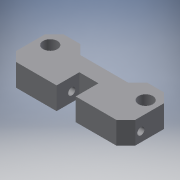
# Autodesk Inventor part: sensor bracket
Saved by Autodesk Inventor 2016 (Build 200138000, 138)
## iProperties
Created: 2016-01-06
Part Number: sensor bracket
Material: Generic
Document SubType Name: Modeling
Designer: RMcComber
Density: 1 g/cm^3
Appearance: Default
Author: RMcComber
Autodesk Inventor part; units mm, degrees
ref_plane "YZ Plane" through (0, 0, 0) normal (1, 0, 0) x (0, 1, 0)
ref_plane "XZ Plane" through (0, 0, 0) normal (0, 1, 0) x (-1, 0, 0)
ref_plane "XY Plane" through (0, 0, 0) normal (0, 0, 1) x (1, 0, 0)
sketch "Sketch1" plane through (0, 0, 0) normal (0, 0, 1) x (1, 0, 0)
  line L0 (0, 0) -> (60, 0) construction
  circle A0 centre (0, 0) radius 4.5
  circle A1 centre (60, 0) radius 4.5
  line L1 (67.5, -20) -> (-7.5, -20)
  line L2 (-7.5, -20) -> (-7.5, 20)
  line L3 (-7.5, 20) -> (67.5, 20)
  line L4 (67.5, 20) -> (67.5, -20)
  line L5 (67.5, -20) -> (-7.5, 20) construction
  line L6 (-7.5, -20) -> (67.5, 20) construction
  point P0 (30, 0)
  dimension "d0" = 9
  dimension "d1" = 60
  dimension "d2" = 40
  dimension "d3" = 75
  constraints: 14 end point, 3 midpoint, 2 centre point, 2 coincident, 2 horizontal, 2 parallel, 1 equal radius, 1 perpendicular
  measures "d0" diameter of A0
  measures "d1" distance of L0.start L0.end
  measures "d2" distance of L1.end L2.end
  measures "d3" distance of L2.end L3.end
extrude "Extrusion1" add sketch "Sketch1" along normal blind 14
sketch "Sketch2" plane through (0, 0, 14) normal (0, 0, 1) x (1, 0, 0)
  line L0 (-7.5, -20) -> (67.5, -20) projected
  line L1 (24, -20) -> (36, -20)
  line L2 (36, -20) -> (36, -5.7)
  line L3 (36, -5.7) -> (24, -5.7)
  line L4 (24, -5.7) -> (24, -20)
  point P0 (30, -20)
  dimension "d6" = 12
  dimension "d7" = 14.3
  constraints: 8 end point, 2 midpoint, 2 parallel, 1 horizontal, 1 perpendicular
  measures "d6" distance of L2.end L3.end
  measures "d7" distance of L3.end L1.start
extrude "Extrusion2" cut sketch "Sketch2" against normal through all
sketch "Sketch3" plane through (24, -20, 14) normal (1, 0, 0) x (0, 0, -1)
  line L0 (0, 0) -> (8, 0) construction
  line L1 (8, 0) -> (8, 9.5) construction
  line L2 (8, 9.5) -> (0, 9.5) construction
  line L3 (0, 9.5) -> (0, 0) construction
  circle A0 centre (8, 9.5) radius 2.25
  point P0 (14, 20)
  dimension "d10" = 8
  dimension "d11" = 9.5
  dimension "d12" = 4.5
  constraints: 8 end point, 2 parallel, 1 centre point, 1 coincident, 1 horizontal, 1 perpendicular
  measures "d10" distance of L1.end L2.end
  measures "d11" distance of L0.end L1.end
  measures "d12" diameter of A0
extrude "Extrusion3" cut sketch "Sketch3" along normal through all both and the other way through all
sketch "Sketch4" plane through (0, 0, 14) normal (0, 0, 1) x (1, 0, 0)
  line L0 (67.5, -20) -> (67.5, 20) projected
  circle A0 centre (0, 0) radius 4.5 projected
  line L1 (-7.5, 20) -> (67.5, 20)
  line L2 (67.5, 20) -> (67.5, 10)
  line L3 (67.5, 10) -> (-7.5, 10)
  line L4 (-7.5, 10) -> (-7.5, 20)
  dimension "d15" = 10
  constraints: 8 end point, 2 parallel, 1 horizontal, 1 perpendicular, 1 point on line
  measures "d15" distance from line of A0.centre L3
extrude "Extrusion4" cut sketch "Sketch4" against normal through all contours L3 L4 L1 L0
sketch "Sketch5" plane through (0, 0, 0) normal (0, 0, -1) x (-1, 0, 0)
  line L0 (7.5, 10) -> (-67.5, 10) projected
  line L1 (-45, 10) -> (-15, 10)
  line L2 (-15, 10) -> (-15, 4)
  line L3 (-15, 4) -> (-45, 4)
  line L4 (-45, 4) -> (-45, 10)
  point P0 (-30, 10)
  dimension "d18" = 30
  dimension "d19" = 6
  constraints: 8 end point, 2 midpoint, 2 parallel, 1 horizontal, 1 perpendicular
  measures "d18" distance of L2.end L3.end
  measures "d19" distance of L3.end L1.start
extrude "Extrusion5" cut sketch "Sketch5" against normal through all
chamfer "Chamfer1" distance 6 angle 45 2 edges at (45, 10, 7) (15, 10, 7)
chamfer "Chamfer2" distance 6 angle 45 4 edges at (-7.5, 10, 7) (67.5, 10, 7) (-7.5, -20, 7) (67.5, -20, 7)
body "Solid1"
